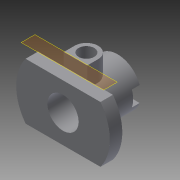
# Autodesk Inventor part: 第一次上机-模型3（改）
Saved by Autodesk Inventor 2013 (Build 170138000, 138)
## iProperties
Created: 2016-11-06
Part Number: 第一次上机-模型3（改）
Material: 常规
Document SubType Name: Modeling
Designer: Administrator
Density: 1 g/cm^3
Author: Administrator
Autodesk Inventor part; units mm, degrees
note: some values were not read from the file. Chosen so that the rebuilt part matches the saved one: direction of "孔2".
ref_plane "YZ Plane" through (0, 0, 0) normal (1, 0, 0) x (0, 1, 0)
ref_plane "XZ Plane" through (0, 0, 0) normal (0, 1, 0) x (-1, 0, 0)
ref_plane "XY Plane" through (0, 0, 0) normal (0, 0, 1) x (1, 0, 0)
sketch "草图1" plane through (0, 0, 0) normal (0, 1, 0) x (-1, 0, 0)
  line L0 (-24, 18) -> (24, 18)
  line L1 (24, 0) -> (39.8795, 0) construction
  line L2 (-24, -18) -> (24, -18)
  arc A0 (-24, 18) -> (-24, -18) centre (0, 0) ccw
  arc A1 (24, -18) -> (24, 18) centre (0, 0) ccw
  dimension "d9" = 18
  dimension "d10" = 30
  constraints: 6 end point, 4 point on circle, 2 centre point, 2 symmetric about line, 1 coincident, 1 concentric, 1 horizontal, 1 parallel
  measures "d9" distance from line of point (0, 0) L0
  measures "d10" radius of A1
extrude "拉伸1" add sketch "草图1" along normal blind 8
sketch "草图2" plane through (0, 8, 0) normal (0, 1, 0) x (1, 0, 0)
  arc A0 (-24, 18) -> (-24, -18) centre (0, 0) ccw projected
  circle A1 centre (0, 0) radius 15
  dimension "d13" = 30
  constraints: 1 centre point, 1 coincident
  measures "d13" diameter of A1
extrude "拉伸2" add sketch "草图2" along normal blind 27
hole "孔1" at (0, 35, 0) direction (0, -1, 0) diameter 20 end through all
ref_plane "工作平面1" through (-24, 0, 26) normal (0, 0, 1) x (1, 0, 0)
sketch "草图3" plane through (-24, 0, 26) normal (0, 0, 1) x (1, 0, 0)
  line L0 (0, 8) -> (48, 8) projected
  line L1 (16.5, 8) -> (16.5, 15)
  arc A0 (31.5, 15) -> (16.5, 15) centre (24, 15) ccw
  line L2 (31.5, 15) -> (31.5, 8)
  point P0 (24, 0)
  dimension "d27" = 7
  dimension "d29" = 7.5
  constraints: 4 end point, 2 perpendicular, 2 point on circle, 2 point on line, 2 tangent, 1 centre point, 1 vertical alignment
  measures "d27" distance of L1.start L1.end
  measures "d29" radius of A0
extrude "拉伸3" add sketch "草图3" against normal up to surface
hole "孔2" at (0, 15, 26) direction (0, 0, -1) diameter 10 end up to surface
sketch "草图4" plane through (0, 0, 0) normal (1, 0, 0) x (0, 1, 0)
  line L0 (35, 10) -> (35, -10) projected
  line L1 (30, 5) -> (35, 5)
  line L2 (35, 5) -> (35, -5)
  line L3 (35, -5) -> (30, -5)
  line L4 (30, -5) -> (30, 5)
  line L5 (6.6641, 0) -> (11.8794, 0) construction
  point P0 (0, 0)
  dimension "d41" = 5
  dimension "d43" = 10
  constraints: 10 end point, 2 parallel, 2 perpendicular, 2 point on line, 1 horizontal, 1 other
  measures "d41" distance of L2.end L3.end
  measures "d43" distance between parallel lines of L3 L1
extrude "拉伸4" cut sketch "草图4" along normal through all both and the other way through all
